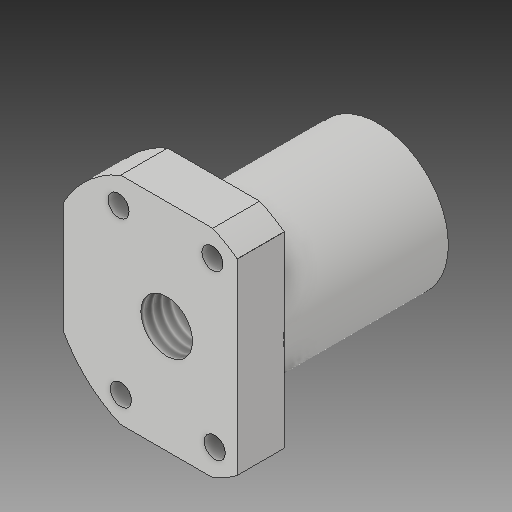
# Autodesk Inventor part: nut
Saved by Autodesk Inventor 2018 (Build 220112000, 112)
## iProperties
Created: 2017-06-20
Part Number: nut
Material: Generic
Document SubType Name: Modeling
Designer: M228544
Density: 1 g/cm^3
Appearance: Default
Mass: 35.244 g
Surface Area: 98.5967 cm^2
Volume: 35.244 cm^3
Author: M228544
Autodesk Inventor part; units mm, degrees
ref_plane "YZ Plane" through (0, 0, 0) normal (1, 0, 0) x (0, 1, 0)
ref_plane "XZ Plane" through (0, 0, 0) normal (0, 1, 0) x (-1, 0, 0)
sketch "Sketch1" plane through (0, 0, 0) normal (0, 1, 0) x (-1, 0, 0)
  line L0 (0, 0) -> (-25, 0)
  line L1 (-25, 0) -> (-25, -10)
  line L2 (-25, -10) -> (-15, -10)
  line L3 (-15, -10) -> (-15, -45)
  line L4 (-15, -45) -> (0, -45)
  line L5 (0, 0) -> (0, -45)
  dimension "d3" = 25
  dimension "d4" = 10
  dimension "d5" = 10
  dimension "d6" = 35
  dimension "d7" = 15
  constraints: 12 end point, 4 perpendicular, 1 horizontal
  measures "d3" distance of L0.start L0.end
  measures "d4" distance of L0.end L1.end
  measures "d5" distance of L1.end L2.end
  measures "d6" distance of L2.end L3.end
  measures "d7" distance of L3.end L4.end
revolve "Revolution1" add sketch "Sketch1" angle 360 about axis through (0, 0, 0) along (0, 0, -1)
sketch "Sketch2" plane through (0, 0, 0) normal (0, 0, 1) x (1, 0, 0)
  line L0 (0, 0) -> (30.242, 0) construction
  line L1 (0, 0.5707) -> (22.435, 0.5707) construction
  circle A0 centre (9.7519, 17.4614) radius 2.25
  circle A1 centre (19.998, 0.2854) radius 2.25
  circle A2 centre (10.2461, -17.1761) radius 2.25
  circle A3 centre (-9.7519, -17.4614) radius 2.25
  circle A4 centre (-19.998, -0.2854) radius 2.25
  circle A5 centre (-10.2461, 17.1761) radius 2.25
  dimension "d12" = 4.5
  dimension "d15" = 360
  constraints: 6 centre point, 4 end point, 2 horizontal, 1 coincident, 13 other
  measures "d12" diameter of A0
extrude "Extrusion1" cut sketch "Sketch2" against normal through all
sketch "Sketch3" plane through (0, 0, 0) normal (0, 0, 1) x (1, 0, 0)
  circle A0 centre (0, 0) radius 5.5
  dimension "d19" = 11
  constraints: 1 centre point, 1 coincident
  measures "d19" diameter of A0
extrude "Extrusion2" cut sketch "Sketch3" against normal through all
thread "Thread1" size "1/2-13 UNC" class "2B" standard "ANSI Unified Screw Threads" full length
sketch "Sketch4" plane through (0, 0, 0) normal (0, 0, 1) x (1, 0, 0)
  circle A0 centre (0, 0) radius 25 projected
  line L0 (-17, 0) -> (-17, 18.3303)
  line L1 (-17, 0) -> (-17, -18.3303)
  constraints: 4 end point, 2 point on circle, 1 point on line
extrude "Extrusion3" cut sketch "Sketch4" against normal blind 15 contours L0 L1 A0 picked at (-18.2676, -10.7318)
ref_plane "Work Plane1" through (-15, 0, -27.5) normal (-1, 0, 0) x (0, -1, 0)
sketch "Sketch5" plane through (-15, 0, -27.5) normal (-1, 0, 0) x (0, -1, 0)
  line L0 (1.9646, 17.5) -> (-2.5354, 17.5) projected
  line L1 (15, -17.5) -> (-15, -17.5) projected
  line L2 (0, -11.5) -> (-5, -11.5)
  line L3 (-5.5, 27.5) -> (-5.5, -17.5) projected
  line L4 (-5, -11.5) -> (-5, 17.5)
  line L5 (15, 17.5) -> (-15, 17.5) projected
  line L6 (0, -11.5) -> (5, -11.5)
  line L7 (5, -11.5) -> (5, 17.5)
  line L8 (5, 17.5) -> (-5, 17.5)
  point P0 (0, 27.5)
  constraints: 10 end point, 3 perpendicular, 2 point on line, 1 collinear, 1 horizontal
extrude "Extrusion4" cut sketch "Sketch5" against normal blind 1
sketch "Sketch9" plane through (0, 0, -10) normal (0, 0, -1) x (-1, 0, 0)
  line L0 (14, 5) -> (14, -5) projected
  line L1 (14, 0) -> (22, 0)
  line L2 (22, 0) -> (22, -11.8743)
  line L3 (22, -11.8743) -> (22, 11.8743)
  arc A0 (22, 11.8743) -> (17.2515, 18.0938) centre (0, 0) ccw
  line L4 (17, -18.3303) -> (17, 18.3303) projected
  line L5 (17, 18.3303) -> (17, -18.3303)
  line L6 (17, 18.3303) -> (17, -18.3303) projected
  arc A1 (17, -18.3303) -> (22, -11.8743) centre (0, 0) ccw
  arc A2 (22, 11.8743) -> (17, 18.3303) centre (0, 0) ccw
  arc A3 (14.1421, 5) -> (14.1421, -5) centre (0, 0) ccw projected
  dimension "d59" = 8
  constraints: 8 end point, 6 point on circle, 3 centre point, 1 collinear, 1 horizontal, 1 midpoint, 1 perpendicular, 1 point on line
  measures "d59" distance of L1.start L1.end
extrude "Extrusion5" add sketch "Sketch9" against normal blind 10
sketch "Sketch20" plane through (-14, 0, -27.5) normal (-1, 0, 0) x (0, 0, 1)
  line L0 (17.5, -11.8743) -> (17.5, 11.8743) projected
  circle A0 centre (11.5, 9.25) radius 3.75
  line L1 (-17.5, -15) -> (-17.5, 15) projected
  line L2 (11.5, 9.25) -> (-3.7889, -9.25)
  circle A1 centre (-3.7889, -9.25) radius 3.75
  point P0 (27.5, 0)
  dimension "d85" = 7.5
  dimension "d87" = 24
  dimension "d88" = 7.5
  constraints: 2 centre point, 2 end point, 1 coincident
  measures "d85" diameter of A0
  measures "d87" distance of L2.start L2.end
  measures "d88" diameter of A1
extrude "Extrusion8" cut sketch "Sketch20" against normal blind 4.75
sketch "Sketch21" plane through (-22, -11.8743, -10) normal (0, 0, -1) x (-1, 0, 0)
  point P0 (-22, 11.8743)
sketch "Sketch22" plane through (-22, -11.8743, -10) normal (0, 0, -1) x (-1, 0, 0)
  point P0 (-22, 11.8743)
sketch "Sketch23" plane through (-22, -11.8743, -10) normal (0, 0, -1) x (-1, 0, 0)
  arc A0 (-7.8579, 16.8743) -> (-7.8579, 6.8743) centre (-22, 11.8743) ccw projected
  arc A1 (0, 23.7487) -> (0, 0) centre (-22, 11.8743) ccw projected
  line L0 (-37, -8.1257) -> (-47.4738, -8.1257)
  line L1 (-47.4738, -8.1257) -> (-47.4738, 31.8346)
  line L2 (-47.4738, 31.8346) -> (-37, 31.8346)
  line L3 (-37, 31.8346) -> (-37, -8.1257)
  line L4 (-22, -13.1257) -> (-22, -11.1257) construction
  line L5 (-31.798, -11.1257) -> (-12.0273, -11.1257)
  line L6 (-12.0273, -11.1257) -> (-12.0273, -17.6927)
  line L7 (-12.0273, -17.6927) -> (-31.798, -17.6927)
  line L8 (-31.798, -17.6927) -> (-31.798, -11.1257)
  line L9 (-22, 11.8743) -> (-7, 11.8743) construction
  line L10 (-31.798, 34.8743) -> (-12.0273, 34.8743)
  line L11 (-12.0273, 34.8743) -> (-12.0273, 41.4414)
  line L12 (-12.0273, 41.4414) -> (-31.798, 41.4414)
  line L13 (-31.798, 41.4414) -> (-31.798, 34.8743)
  dimension "d91" = 2
  constraints: 28 end point, 4 parallel, 4 symmetric about line, 3 horizontal, 3 point on circle, 2 perpendicular, 1 vertical
  measures "d91" distance of L4.start L4.end
extrude "Extrusion9" cut sketch "Sketch23" against normal blind 10
body "Solid1"
